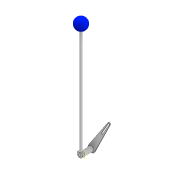
# Autodesk Inventor part: Palanca
Saved by Autodesk Inventor 2021 (Build 250183000, 183)
## iProperties
Created: 2021-04-19
Part Number: Palanca
Material: Genérico
Document SubType Name: Modeling
Designer: carlo
Density: 1 g/cm^3
Appearance: Valor por defecto
Author: carlo
Autodesk Inventor part; units mm, degrees
ref_plane "YZ Plane" through (0, 0, 0) normal (1, 0, 0) x (0, 1, 0)
ref_plane "XZ Plane" through (0, 0, 0) normal (0, 1, 0) x (-1, 0, 0)
ref_plane "XY Plane" through (0, 0, 0) normal (0, 0, 1) x (1, 0, 0)
ref_plane "Plano de trabajo1" through (0, 0, 0) normal (0, 0, -1) x (-1, 0, 0)
sketch "Boceto4" plane through (0, 0, 0) normal (0, 0, -1) x (-1, 0, 0)
  circle A0 centre (0, 0) radius 5
  circle A1 centre (0, 0) radius 10
  dimension "d16" = 20
  constraints: 2 centre point, 2 coincident
  measures "d16" diameter of A1
extrude "Extrusión2" add sketch "Boceto4" along normal blind 40
sketch "Boceto5" plane through (0, 0, -40) normal (0, 0, -1) x (-1, 0, 0)
  arc A0 (-15, 0) -> (15, 0) centre (0, 0) ccw projected
  line L0 (-72.8349, 131.1538) -> (-42.8349, 79.1923)
  line L1 (-47.1651, 76.6923) -> (-77.1651, 128.6538)
  arc A1 (-72.8349, 131.1538) -> (-77.1651, 128.6538) centre (-75, 129.9038) ccw
  arc A2 (-70.4175, 131.9041) -> (-79.3301, 127.4038) centre (-75, 129.9038) ccw
  arc A3 (-47.1651, 76.6923) -> (-42.8349, 79.1923) centre (-45, 77.9423) ccw
  arc A4 (-15, 0) -> (15, 0) centre (0, 0) ccw
  arc A5 (-13.6856, -6.1404) -> (12.4137, 8.4202) centre (0, 0) ccw
  line L2 (-79.3301, 127.4038) -> (-13.2209, -7.0857)
  line L3 (-70.4175, 131.9041) -> (12.5, 8.2916)
  circle A6 centre (0, 0) radius 5
  point P0 (-13.2209, -7.0857)
  point P1 (15, 0)
  point P2 (12.5, 8.2916)
  constraints: 12 point on circle, 8 end point, 6 centre point, 2 coincident, 2 point on line
extrude "Extrusión3" add sketch "Boceto5" along normal blind 3 contours L2 A2 L3 A5 A0
sketch "Boceto10" plane through (0, 0, 0) normal (0, 0, -1) x (-1, 0, 0)
  arc A0 (-10, 0) -> (10, 0) centre (0, 0) ccw
  circle A1 centre (0, 0) radius 10 projected
  line L0 (-10, 0) -> (-10, 10)
  line L1 (-10, 10) -> (10, 10)
  line L2 (10, 10) -> (10, 0)
  circle A2 centre (0, 0) radius 5
  dimension "d29" = 10
  constraints: 6 end point, 2 centre point, 2 coincident, 2 point on circle, 1 horizontal alignment, 1 parallel, 1 other
  measures "d29" diameter of A2
extrude "Extrusión5" add sketch "Boceto10" against normal blind 10
sketch "Boceto11" plane through (-10, 10, 0) normal (0, 1, 0) x (1, 0, 0)
  circle A0 centre (10, -5) radius 5
  point P0 (10, 0)
  constraints: 1 centre point
extrude "Extrusión6" add sketch "Boceto11" along normal blind 480
sketch "Boceto12" plane through (0, 490, 5) normal (0, 1, 0) x (1, 0, 0)
  arc A0 (25, 0) -> (-25, 0) centre (0, 0) ccw
  line L0 (25, 0) -> (-25, 0)
  point P0 (0, 5)
  constraints: 2 end point, 2 point on circle, 1 centre point, 1 horizontal
revolve "Revolución1" add sketch "Boceto12" angle 360 about axis through (25, 490, 5) along (-1, 0, 0)
